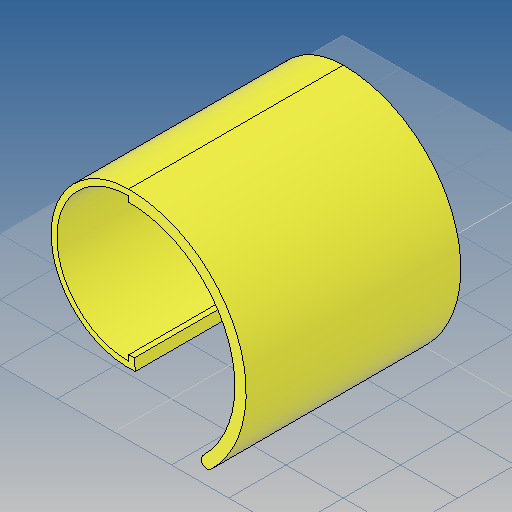
# Autodesk Inventor part: Züklon_Lufteinlass
Saved by Autodesk Inventor 2019 (Build 230136000, 136)
## iProperties
Created: 2020-08-01
Part Number: Züklon_Lufteinlass
Material: Generisch
Document SubType Name: Modeling
Designer: Stefan
Mass: 40.7918 g
Surface Area: 286.235 cm^2
Volume: 40.7918 cm^3
Density: 1 g/cm^3
Appearance: Glatt - Gelb
Author: Stefan
Autodesk Inventor part; units mm, degrees
ref_plane "YZ Plane" through (0, 0, 0) normal (1, 0, 0) x (0, 1, 0)
ref_plane "XZ Plane" through (0, 0, 0) normal (0, 1, 0) x (-1, 0, 0)
ref_plane "XY Plane" through (0, 0, 0) normal (0, 0, 1) x (1, 0, 0)
sketch "Skizze1" plane through (0, 0, 0) normal (0, 0, 1) x (1, 0, 0)
  circle A0 centre (0, 0) radius 25.05 construction
  arc A1 (28.7396, -43.3579) -> (0, 27.05) centre (0, -14.0195) ccw
  circle A2 centre (0, 0) radius 23.1 construction
  line L0 (0, 25.05) -> (0, 23.1)
  arc A3 (25.9755, -40.5362) -> (0, 23.1) centre (0, -14.0195) ccw
  line L1 (0, -63.4548) -> (0, 53.3986) construction
  line L2 (0, -25.05) -> (0, -23.1)
  line L3 (2.0133, -23.0121) -> (2.3576, -26.9471)
  arc A4 (0, 27.05) -> (2.3576, -26.9471) centre (0, 0) ccw
  arc A5 (0, -23.1) -> (2.0133, -23.0121) centre (0, 0) ccw
  arc A6 (0, 25.05) -> (0, -25.05) centre (0, 0) ccw
  arc A7 (25.9755, -40.5362) -> (28.7396, -43.3579) centre (27.3576, -41.9471) ccw
  arc A8 (3.0076, -22.9034) -> (0, 23.1) centre (0, 0) ccw
  line L4 (3.0076, -22.9034) -> (3.3521, -26.8415)
  circle A9 centre (0, 0) radius 27.05 construction
  arc A10 (25.4302, -42.3783) -> (3.3521, -26.8415) centre (5.8399, -46.7614) ccw
  dimension "d0" = 50.1
  dimension "d2" = 46.2
  dimension "d3" = 2
  dimension "d4" = 5
  dimension "d11" = 25
  dimension "d12" = 15
  dimension "d16" = 1
  constraints: 24 point on circle, 11 centre point, 8 end point, 6 tangent, 5 concentric, 3 coincident, 3 point on line, 1 line through centre, 1 parallel, 1 vertical
  measures "d0" diameter of A0
  measures "d2" diameter of A2
  measures "d3" radial gap between concentric circles of A0 A4
  measures "d4" angle of L3 L2
  measures "d11" horizontal distance of A7.centre L3.end
  measures "d12" vertical distance of A7.centre L3.end
  measures "d16" distance between parallel lines of L3 L4
extrude "Extrusion1" add sketch "Skizze1" along normal blind 75 contours A7 A3 L0 A6 L2 A5 L3 A4 A1
equation "\"d0\" = ht_diameter + gap_fit"
equation "\"d2\" = ht_diameter - 2 * ht_thickness"
equation "\"kg_thickness\" = 4.9"
equation "\"ht_diameter\" = 50"
equation "\"ht_thickness\" = 1.9"
equation "\"case_thickness\" = 18"
equation "\"gap_fit\" = 0.1"
equation "\"gap_slide\" = 0.2"
equation "\"gap_air\" = 1"
equation "\"bore_diameter\" = 73"
equation "\"tape_thickness\" = 3"
equation "\"tape_width\" = 15"
equation "\"mdf_thickness\" = 6"
equation "\"inner_thickness\" = 15"
equation "\"inner_depth\" = 255"
